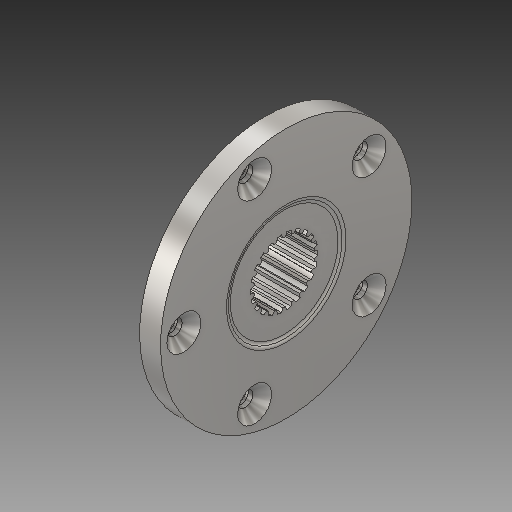
# Autodesk Inventor part: 332-07
Saved by Autodesk Inventor 2019 (Build 230136000, 136)
## iProperties
Company: Autodesk Inc.
Created: 2017-03-14
Part Number: 332-07
Material: Stainless Steel
Document SubType Name: Modeling
Designer: Autodesk Inc.
Density: 8 g/cm^3
Appearance: Semi-Polished
Mass: 719.286 g
Surface Area: 266.868 cm^2
Volume: 89.9108 cm^3
Author: Inventor
Autodesk Inventor part; units mm, degrees
ref_plane "YZ Plane" through (0, 0, 0) normal (1, 0, 0) x (0, 1, 0)
ref_plane "XZ Plane" through (0, 0, 0) normal (0, 1, 0) x (-1, 0, 0)
ref_plane "XY Plane" through (0, 0, 0) normal (0, 0, 1) x (1, 0, 0)
sketch "Sketch1" plane through (0, 0, 0) normal (1, 0, 0) x (0, 1, 0)
  circle A0 centre (0, 0) radius 54
  circle A1 centre (0, 0) radius 21.5
  circle A2 centre (25.8626, -35.5967) radius 3.3 projected
  circle A3 centre (0, 0) radius 12.5
  arc A4 (12.7803, 6.8493) -> (11.5395, 8.7801) centre (0, 0) ccw
  line L0 (13, 0.5) -> (13, -0.5)
  line L1 (13, 0.5) -> (14.4545, 1.1476)
  line L2 (13, -0.5) -> (14.4545, -1.1476)
  line L3 (12.3325, 4.1423) -> (13.5457, 5.1734)
  line L4 (12.3325, 4.1423) -> (12.6143, 3.1828)
  line L5 (12.6143, 3.1828) -> (14.1923, 2.9712)
  line L6 (10.666, 7.449) -> (11.5395, 8.7801)
  line L7 (10.666, 7.449) -> (11.2066, 6.6077)
  line L8 (11.2066, 6.6077) -> (12.7803, 6.8493)
  line L9 (8.1353, 10.1522) -> (8.5984, 11.6755)
  line L10 (8.1353, 10.1522) -> (8.8911, 9.4973)
  line L11 (8.8911, 9.4973) -> (10.333, 10.1725)
  line L12 (4.9456, 12.0329) -> (4.9607, 13.625)
  line L13 (4.9456, 12.0329) -> (5.8552, 11.6175)
  line L14 (5.8552, 11.6175) -> (7.0485, 12.6716)
  line L15 (1.3552, 12.9388) -> (0.9212, 14.4707)
  line L16 (1.3552, 12.9388) -> (2.345, 12.7965)
  line L17 (2.345, 12.7965) -> (3.193, 14.1441)
  line L18 (-2.345, 12.7965) -> (-3.193, 14.1441)
  line L19 (-2.345, 12.7965) -> (-1.3552, 12.9388)
  line L20 (-1.3552, 12.9388) -> (-0.9212, 14.4707)
  line L21 (-5.8552, 11.6175) -> (-7.0485, 12.6716)
  line L22 (-5.8552, 11.6175) -> (-4.9456, 12.0329)
  line L23 (-4.9456, 12.0329) -> (-4.9607, 13.625)
  line L24 (-8.8911, 9.4973) -> (-10.333, 10.1725)
  line L25 (-8.8911, 9.4973) -> (-8.1353, 10.1522)
  line L26 (-8.1353, 10.1522) -> (-8.5984, 11.6755)
  line L27 (-11.2066, 6.6077) -> (-12.7803, 6.8493)
  line L28 (-11.2066, 6.6077) -> (-10.666, 7.449)
  line L29 (-10.666, 7.449) -> (-11.5395, 8.7801)
  line L30 (-12.6143, 3.1828) -> (-14.1923, 2.9712)
  line L31 (-12.6143, 3.1828) -> (-12.3325, 4.1423)
  line L32 (-12.3325, 4.1423) -> (-13.5457, 5.1734)
  line L33 (-13, -0.5) -> (-14.4545, -1.1476)
  line L34 (-13, -0.5) -> (-13, 0.5)
  line L35 (-13, 0.5) -> (-14.4545, 1.1476)
  line L36 (-12.3325, -4.1423) -> (-13.5457, -5.1734)
  line L37 (-12.3325, -4.1423) -> (-12.6143, -3.1828)
  line L38 (-12.6143, -3.1828) -> (-14.1923, -2.9712)
  line L39 (-10.666, -7.449) -> (-11.5395, -8.7801)
  line L40 (-10.666, -7.449) -> (-11.2066, -6.6077)
  line L41 (-11.2066, -6.6077) -> (-12.7803, -6.8493)
  line L42 (-8.1353, -10.1522) -> (-8.5984, -11.6755)
  line L43 (-8.1353, -10.1522) -> (-8.8911, -9.4973)
  line L44 (-8.8911, -9.4973) -> (-10.333, -10.1725)
  line L45 (-4.9456, -12.0329) -> (-4.9607, -13.625)
  line L46 (-4.9456, -12.0329) -> (-5.8552, -11.6175)
  line L47 (-5.8552, -11.6175) -> (-7.0485, -12.6716)
  line L48 (-1.3552, -12.9388) -> (-0.9212, -14.4707)
  line L49 (-1.3552, -12.9388) -> (-2.345, -12.7965)
  line L50 (-2.345, -12.7965) -> (-3.193, -14.1441)
  line L51 (2.345, -12.7965) -> (3.193, -14.1441)
  line L52 (2.345, -12.7965) -> (1.3552, -12.9388)
  line L53 (1.3552, -12.9388) -> (0.9212, -14.4707)
  line L54 (5.8552, -11.6175) -> (7.0485, -12.6716)
  line L55 (5.8552, -11.6175) -> (4.9456, -12.0329)
  line L56 (4.9456, -12.0329) -> (4.9607, -13.625)
  line L57 (8.8911, -9.4973) -> (10.333, -10.1725)
  line L58 (8.8911, -9.4973) -> (8.1353, -10.1522)
  line L59 (8.1353, -10.1522) -> (8.5984, -11.6755)
  line L60 (11.2066, -6.6077) -> (12.7803, -6.8493)
  line L61 (11.2066, -6.6077) -> (10.666, -7.449)
  line L62 (10.666, -7.449) -> (11.5395, -8.7801)
  line L63 (12.6143, -3.1828) -> (14.1923, -2.9712)
  line L64 (12.6143, -3.1828) -> (12.3325, -4.1423)
  line L65 (12.3325, -4.1423) -> (13.5457, -5.1734)
  arc A5 (13.5457, 5.1734) -> (12.7803, 6.8493) centre (0, 0) ccw
  arc A6 (14.1923, 2.9712) -> (13.5457, 5.1734) centre (0, 0) ccw
  arc A7 (14.4545, 1.1476) -> (14.1923, 2.9712) centre (0, 0) ccw
  arc A8 (14.4545, -1.1476) -> (14.4545, 1.1476) centre (0, 0) ccw
  arc A9 (14.1923, -2.9712) -> (14.4545, -1.1476) centre (0, 0) ccw
  arc A10 (13.5457, -5.1734) -> (14.1923, -2.9712) centre (0, 0) ccw
  arc A11 (12.7803, -6.8493) -> (13.5457, -5.1734) centre (0, 0) ccw
  arc A12 (11.5395, -8.7801) -> (12.7803, -6.8493) centre (0, 0) ccw
  arc A13 (10.333, -10.1725) -> (11.5395, -8.7801) centre (0, 0) ccw
  arc A14 (8.5984, -11.6755) -> (10.333, -10.1725) centre (0, 0) ccw
  arc A15 (7.0485, -12.6716) -> (8.5984, -11.6755) centre (0, 0) ccw
  arc A16 (4.9607, -13.625) -> (7.0485, -12.6716) centre (0, 0) ccw
  arc A17 (3.193, -14.1441) -> (4.9607, -13.625) centre (0, 0) ccw
  arc A18 (0.9212, -14.4707) -> (3.193, -14.1441) centre (0, 0) ccw
  arc A19 (-0.9212, -14.4707) -> (0.9212, -14.4707) centre (0, 0) ccw
  arc A20 (-3.193, -14.1441) -> (-0.9212, -14.4707) centre (0, 0) ccw
  arc A21 (-4.9607, -13.625) -> (-3.193, -14.1441) centre (0, 0) ccw
  arc A22 (-7.0485, -12.6716) -> (-4.9607, -13.625) centre (0, 0) ccw
  arc A23 (-8.5984, -11.6755) -> (-7.0485, -12.6716) centre (0, 0) ccw
  arc A24 (-10.333, -10.1725) -> (-8.5984, -11.6755) centre (0, 0) ccw
  arc A25 (-11.5395, -8.7801) -> (-10.333, -10.1725) centre (0, 0) ccw
  arc A26 (-12.7803, -6.8493) -> (-11.5395, -8.7801) centre (0, 0) ccw
  arc A27 (-13.5457, -5.1734) -> (-12.7803, -6.8493) centre (0, 0) ccw
  arc A28 (-14.1923, -2.9712) -> (-13.5457, -5.1734) centre (0, 0) ccw
  arc A29 (-14.4545, -1.1476) -> (-14.1923, -2.9712) centre (0, 0) ccw
  arc A30 (-14.4545, 1.1476) -> (-14.4545, -1.1476) centre (0, 0) ccw
  arc A31 (-14.1923, 2.9712) -> (-14.4545, 1.1476) centre (0, 0) ccw
  arc A32 (-13.5457, 5.1734) -> (-14.1923, 2.9712) centre (0, 0) ccw
  arc A33 (-12.7803, 6.8493) -> (-13.5457, 5.1734) centre (0, 0) ccw
  arc A34 (-11.5395, 8.7801) -> (-12.7803, 6.8493) centre (0, 0) ccw
  arc A35 (-10.333, 10.1725) -> (-11.5395, 8.7801) centre (0, 0) ccw
  arc A36 (-8.5984, 11.6755) -> (-10.333, 10.1725) centre (0, 0) ccw
  arc A37 (-7.0485, 12.6716) -> (-8.5984, 11.6755) centre (0, 0) ccw
  arc A38 (-4.9607, 13.625) -> (-7.0485, 12.6716) centre (0, 0) ccw
  arc A39 (-3.193, 14.1441) -> (-4.9607, 13.625) centre (0, 0) ccw
  arc A40 (-0.9212, 14.4707) -> (-3.193, 14.1441) centre (0, 0) ccw
  arc A41 (0.9212, 14.4707) -> (-0.9212, 14.4707) centre (0, 0) ccw
  arc A42 (3.193, 14.1441) -> (0.9212, 14.4707) centre (0, 0) ccw
  arc A43 (4.9607, 13.625) -> (3.193, 14.1441) centre (0, 0) ccw
  arc A44 (7.0485, 12.6716) -> (4.9607, 13.625) centre (0, 0) ccw
  arc A45 (8.5984, 11.6755) -> (7.0485, 12.6716) centre (0, 0) ccw
  arc A46 (10.333, 10.1725) -> (8.5984, 11.6755) centre (0, 0) ccw
  arc A47 (11.5395, 8.7801) -> (10.333, 10.1725) centre (0, 0) ccw
  dimension "d40" = 29
  dimension "d41" = 1
  dimension "d42" = 13
  dimension "d43" = 114
  dimension "d44" = 114
  dimension "d45" = 360
  dimension "d46" = 25
  dimension "d47" = 43
  dimension "d48" = 108
  constraints: 132 end point, 3 centre point, 2 concentric, 2 horizontal alignment, 2 vertical alignment, 1 equal length, 1 vertical, 287 other
  measures "d41" distance of L1.start L0.end
  measures "d42" distance from line of A3.centre L0
  measures "d43" angle of L0 L1
  measures "d44" angle of L0 L2
  measures "d46" diameter of A3
  measures "d47" diameter of A1
  measures "d48" diameter of A0
extrude "Extrusion1" add sketch "Sketch1" along normal mid plane 9 contours A0 | A1 | A2 | A3 | L8 L7 L6 A4 | A5 L3 L4 L5 A7 L1 L0 L2 A9 L63 L64 L65 A11 L60 L61 L62 A13 L57 L58 L59 A15 L54 L55 L56 A17 L51 L52 L53 A19 L48 L49 L50 A21 L45 L46 L47 A23 L42 L43 L44 A25 L39 L40 L41 A27 L36 L37 L38 A29 L33 L34 L35 A31 L30 L31 L32 A33 L27 L28 L29 A35 L24 L25 L26 A37 L21 L22 L23 A39 L18 L19 L20 A41 L15 L16 L17 A43 L12 L13 L14 A45 L9 L10 L11 A47 L6 L7 L8 | A6 L5 L4 L3 | L11 L10 L9 A46 | A8 L2 L0 L1 | L14 L13 L12 A44 | A10 L65 L64 L63 | L17 L16 L15 A42 | A12 L62 L61 L60 | L20 L19 L18 A40 | A14 L59 L58 L57 | L23 L22 L21 A38 | A16 L56 L55 L54 | L26 L25 L24 A36 | A18 L53 L52 L51 | L29 L28 L27 A34 | A20 L50 L49 L48 | L32 L31 L30 A32 | A22 L47 L46 L45 | L35 L34 L33 A30 | A24 L44 L43 L42 | L38 L37 L36 A28 | A26 L41 L40 L39
sketch "Sketch2" plane through (-4.5, 0, 0) normal (-1, 0, 0) x (0, 0, 1)
  circle A0 centre (0, 0) radius 23
  dimension "d5" = 46
  constraints: 1 centre point, 1 coincident
  measures "d5" diameter of A0
extrude "Extrusion2" add sketch "Sketch2" along normal blind 17
extrude "Extrusion3" cut sketch "Sketch1" along normal through all both and the other way through all contours A3 | A5 L3 L4 L5 A7 L1 L0 L2 A9 L63 L64 L65 A11 L60 L61 L62 A13 L57 L58 L59 A15 L54 L55 L56 A17 L51 L52 L53 A19 L48 L49 L50 A21 L45 L46 L47 A23 L42 L43 L44 A25 L39 L40 L41 A27 L36 L37 L38 A29 L33 L34 L35 A31 L30 L31 L32 A33 L27 L28 L29 A35 L24 L25 L26 A37 L21 L22 L23 A39 L18 L19 L20 A41 L15 L16 L17 A43 L12 L13 L14 A45 L9 L10 L11 A47 L6 L7 L8
hole "Hole1" at (4.5, 0, 0) direction (-1, 0, 0) diameter 48 depth 0.9
fillet "Fillet1" radius 2 1 edges at (4.5, 0, 24)
fillet "Fillet2" radius 2 1 edges at (3.6, 0, 24)
extrude "Extrusion4" cut sketch "Sketch1" along normal through all both and the other way through all contours A2
hole "Hole2" at (-4.5, 25.8626, -35.5967) direction (1, 0, 0) diameter 6.6 end through all counterbore diameter 12 counterbore depth 3
pattern_circular "Circular Pattern1" count 5 over 360 about axis through (-4.5, 0, 0) along (-1, 0, 0) of "Hole2", "Extrusion4"
chamfer "Chamfer1" distance 4 angle 45 10 edges at (4.5, 23.5291, -37.9302) (4.5, 28.196, -33.2633) (4.5, -28.8029, -34.0986) (4.5, -22.9222, -37.0949) (4.5, 43.3447, 10.6564) (4.5, 40.3483, 16.5371) (4.5, -41.3303, 16.8561) (4.5, -42.3627, 10.3374) (4.5, 3.2594, 44.5162) (4.5, -3.2594, 43.4838)
body "Solid1"
